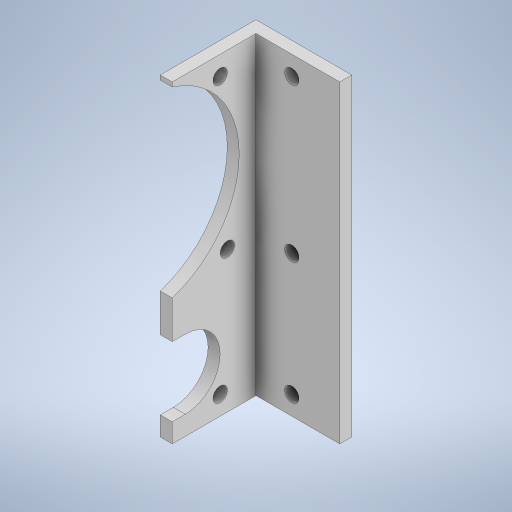
# Autodesk Inventor part: Frame L Branket Opposite Side
Saved by Autodesk Inventor 2023 (Build 270158000, 158)
## iProperties
Created: 2022-12-23
Part Number: Frame L Branket Opposite Side
Material: Generic
Document SubType Name: Modeling
Designer: tgr41
Density: 1 g/cm^3
Appearance: Default
Author: tgr41
Autodesk Inventor part; units mm, degrees
ref_plane "YZ Plane" through (0, 0, 0) normal (1, 0, 0) x (0, 1, 0)
ref_plane "XZ Plane" through (0, 0, 0) normal (0, 1, 0) x (-1, 0, 0)
ref_plane "XY Plane" through (0, 0, 0) normal (0, 0, 1) x (1, 0, 0)
sketch "Sketch1" plane through (0, 0, 0) normal (1, 0, 0) x (0, 1, 0)
  circle A0 centre (5.08, -5.08) radius 1.905
  circle A1 centre (78.105, -5.08) radius 1.905
  circle A2 centre (37.465, -3.175) radius 1.905
  arc A3 (82.0151, -17.78) -> (33.5549, -17.78) centre (57.785, -25.4) ccw
  line L0 (82.0151, -17.78) -> (83.185, -17.78)
  line L1 (83.185, -17.78) -> (83.185, 7.62)
  line L2 (83.185, 7.62) -> (0, 7.62)
  line L3 (0, 7.62) -> (0, -17.78)
  arc A4 (23.495, -14.2875) -> (5.08, -14.2875) centre (14.2875, -14.2875) ccw
  line L4 (82.0151, -17.78) -> (83.185, -17.78)
  line L5 (0, -17.78) -> (5.08, -17.78)
  line L6 (23.495, -17.78) -> (33.5549, -17.78)
  line L7 (23.495, -14.2875) -> (23.495, -17.78)
  line L8 (5.08, -14.2875) -> (5.08, -17.78)
  line L9 (83.185, 7.62) -> (83.185, 4.445)
  line L10 (83.185, 4.445) -> (0, 4.445)
  point P0 (0, 0)
  dimension "d16" = 3.81
  dimension "d41" = 3.175
  dimension "d51" = 3.81
  dimension "d52" = 3.81
  constraints: 22 end point, 7 perpendicular, 5 centre point, 4 point on circle, 2 point on line, 2 tangent
  measures "d16" diameter of A0
  measures "d41" distance of L1.end L9.end
  measures "d51" diameter of A2
  measures "d52" diameter of A1
extrude "Extrusion3" add sketch "Sketch1" along normal blind 3.175 contours A3 L6 L7 A4 L8 L5 L3 L10 L1 L0
extrude "Extrusion4" add sketch "Sketch1" along normal blind 25.4 contours L10 L3 L2 L1
sketch "Sketch3" plane through (0, 0, 7.62) normal (0, 0, 1) x (1, 0, 0)
  line L0 (3.175, 0) -> (25.4, 0) projected
  line L1 (0, 0) -> (25.4, 0)
  line L2 (0, 0) -> (25.4, 0) projected
  line L3 (12.7, 0) -> (12.7, 83.185)
  line L4 (0, 83.185) -> (25.4, 83.185) projected
  circle A0 centre (12.7, 5.08) radius 1.905
  circle A1 centre (12.7, 37.465) radius 1.905
  circle A2 centre (12.7, 78.105) radius 1.905
  dimension "d46" = 3.81
  dimension "d47" = 3.81
  dimension "d48" = 3.81
  constraints: 4 end point, 3 centre point, 3 point on line, 2 midpoint, 1 collinear
  measures "d46" diameter of A0
  measures "d47" diameter of A1
  measures "d48" diameter of A2
extrude "Extrusion5" cut sketch "Sketch3" against normal blind 25.4
mirror "Mirror1" about plane through (0, 23.495, -17.78) normal (0, 0, -1) remove original yes
body "Solid2"
